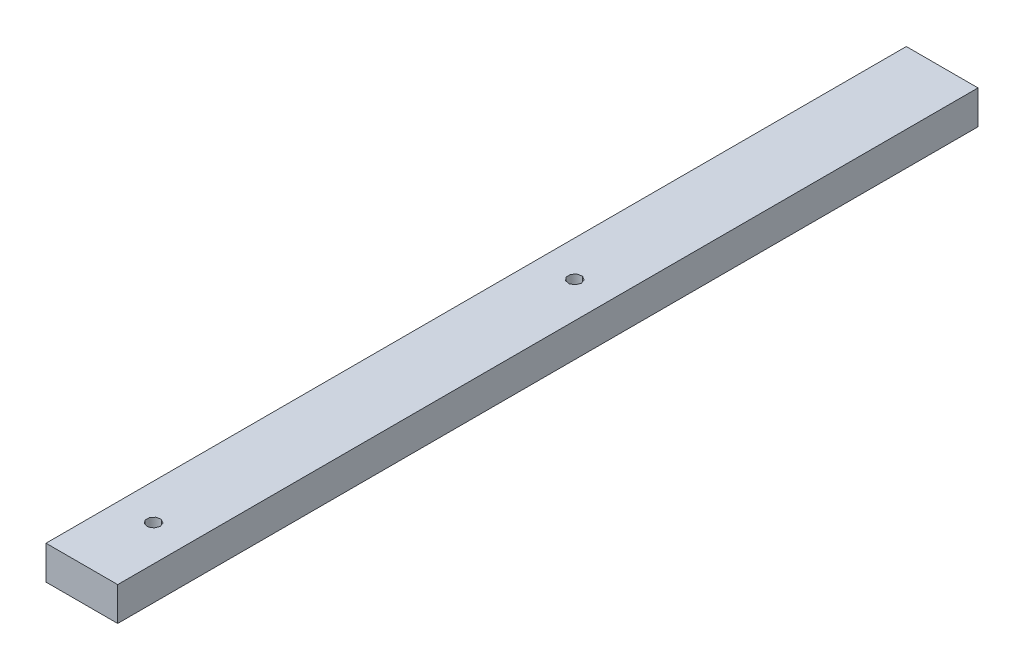
# Autodesk Inventor part: pincer
Saved by Autodesk Inventor 2023 (Build 270158000, 158)
## iProperties
Created: 2023-01-24
Part Number: pincer
Material: Generic
Document SubType Name: Modeling
Designer: Blank Slate
Density: 1 g/cm^3
Appearance: Default
Author: Blank Slate
Autodesk Inventor part; units mm, degrees
ref_plane "YZ Plane" through (0, 0, 0) normal (1, 0, 0) x (0, 1, 0)
ref_plane "XZ Plane" through (0, 0, 0) normal (0, 1, 0) x (-1, 0, 0)
ref_plane "XY Plane" through (0, 0, 0) normal (0, 0, 1) x (1, 0, 0)
sketch "Sketch1" plane through (0, 0, 0) normal (0, 1, 0) x (-1, 0, 0)
  line L0 (0, 0) -> (-25.4, 0)
  line L1 (-25.4, 0) -> (-25.4, -304.8)
  line L2 (-25.4, -304.8) -> (0, -304.8)
  line L3 (0, -304.8) -> (0, 0)
  dimension "d0" = 25.4
  dimension "d1" = 304.8
  constraints: 8 end point, 2 parallel, 1 horizontal, 1 perpendicular
  measures "d0" distance of L2.end L1.end
  measures "d1" distance of L1.end L0.end
extrude "Extrusion1" add sketch "Sketch1" along normal blind 11.938
sketch "Sketch2" plane through (0, 11.938, 0) normal (0, 1, 0) x (1, 0, 0)
  line L0 (0, 0) -> (25.4, 0) projected
  line L1 (12.7, 0) -> (12.7, 304.8) construction
  line L2 (25.4, 304.8) -> (0, 304.8) projected
  line L3 (12.7, 0) -> (12.7, 25.4) construction
  line L4 (12.7, 25.4) -> (0, 25.4) construction
  line L5 (0, 25.4) -> (25.4, 25.4) construction
  line L6 (25.4, 0) -> (25.4, 304.8) construction
  circle A0 centre (12.7, 25.4) radius 2.3813 construction
  line L7 (12.7, 0) -> (12.7, 174.625) construction
  circle A1 centre (12.7, 174.625) radius 2.3812 construction
  dimension "d4" = 25.4
  dimension "d5" = 4.7625
  dimension "d6" = 174.625
  dimension "d7" = 4.7625
  constraints: 10 end point, 4 point on line, 2 centre point, 2 coincident, 2 midpoint, 1 horizontal
  measures "d4" distance of L1.start L3.end
  measures "d5" diameter of A0
  measures "d6" distance of L1.start L7.end
  measures "d7" diameter of A1
hole "Hole1" at (12.7, 11.938, -25.4) at (12.7, 11.938, -174.625) direction (0, -1, 0) diameter 4.7625 end through all
sketch "Sketch3" plane through (0, 0, 0) normal (0, -1, 0) x (1, 0, 0)
  point P0 (0, 0)
body "Solid1"
